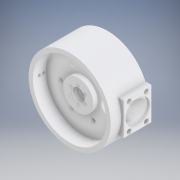
# Autodesk Inventor part: AA036
Saved by Autodesk Inventor 2017 SP1 (Build 210196100, 196)
## iProperties
Created: 2017-10-30
Part Number: AA036
Material: ABS Plastic
Document SubType Name: Modeling
Designer: Zach
Density: 1.06 g/cm^3
Appearance: CR White
Author: Zach
Autodesk Inventor part; units mm, degrees
ref_plane "YZ Plane" through (0, 0, 0) normal (1, 0, 0) x (0, 1, 0)
ref_plane "XZ Plane" through (0, 0, 0) normal (0, 1, 0) x (-1, 0, 0)
ref_plane "XY Plane" through (0, 0, 0) normal (0, 0, 1) x (1, 0, 0)
sketch "Sketch1" plane through (0, 0, 0) normal (0, 0, 1) x (1, 0, 0)
  circle A0 centre (0, 0) radius 47.5
  circle A1 centre (0, 0) radius 4.25
  circle A2 centre (25, 0) radius 2.5
  circle A3 centre (12.5, 21.6506) radius 2.5
  circle A4 centre (-12.5, 21.6506) radius 2.5
  circle A5 centre (-25, 0) radius 2.5
  circle A6 centre (-12.5, -21.6506) radius 2.5
  circle A7 centre (12.5, -21.6506) radius 2.5
  dimension "d0" = 95
  dimension "d1" = 8.5
  dimension "d2" = 5
  dimension "d3" = 25
  dimension "d6" = 360
  constraints: 8 centre point, 2 coincident, 1 horizontal alignment, 13 other
  measures "d0" diameter of A0
  measures "d1" diameter of A1
  measures "d2" diameter of A2
  measures "d3" distance of A2.centre point (0, 0)
extrude "Extrusion1" add sketch "Sketch1" along normal blind 54
ref_plane "Work Plane1" through (0, 0, 16) normal (0, 0, 1) x (1, 0, 0)
sketch "Sketch2" plane through (0, 0, 16) normal (0, 0, 1) x (1, 0, 0)
  circle A0 centre (0, 0) radius 47.5 projected
  line L0 (43.6427, 18.75) -> (50.6427, 18.75)
  line L1 (50.6427, 18.75) -> (50.6427, -18.75)
  line L2 (50.6427, -18.75) -> (43.6427, -18.75)
  line L3 (43.6427, -18.75) -> (43.6427, 18.75)
  point P0 (43.6427, 0)
  dimension "d11" = 7
  dimension "d12" = 37.5
  constraints: 8 end point, 2 parallel, 2 point on circle, 1 horizontal, 1 horizontal alignment, 1 midpoint, 1 perpendicular
  measures "d11" distance of L1.end L2.end
  measures "d12" distance of L0.end L1.end
extrude "Extrusion2" add sketch "Sketch2" along normal mid plane 32 contours A0 L0 L1 L2
sketch "Sketch3" plane through (50.6427, -18.75, 32) normal (1, 0, 0) x (0, 0, -1)
  line L0 (-14, 48.75) -> (46, 48.75)
  line L1 (46, 48.75) -> (46, -11.25)
  line L2 (46, -11.25) -> (-14, -11.25)
  line L3 (-14, -11.25) -> (-14, 48.75)
  line L4 (32, 37.5) -> (0, 37.5) projected
  line L5 (0, 0) -> (0, 37.5) projected
  line L6 (32, 0) -> (0, 0) projected
  line L7 (32, 37.5) -> (32, 0) projected
  line L8 (32, 37.5) -> (32, 0) projected
  point P0 (32, 18.75)
  point P1 (-14, 18.75)
  point P2 (32, 18.75)
  point P3 (16, 48.75)
  point P4 (16, 37.5)
  dimension "d15" = 60
  dimension "d16" = 60
  constraints: 8 end point, 4 midpoint, 2 parallel, 1 horizontal, 1 horizontal alignment, 1 perpendicular, 1 vertical alignment
  measures "d15" distance of L1.end L2.end
  measures "d16" distance of L0.end L1.end
extrude "Extrusion3" add sketch "Sketch3" along normal blind 10 contours L0 L1 L2 L3 | L7 L6 L5 L4
fillet "Fillet1" radius 20 4 edges at (55.6427, 30, 46) (55.6427, 30, -14) (55.6427, -30, -14) (55.6427, -30, 46)
sketch "Sketch4" plane through (60.6427, -18.75, 32) normal (1, 0, 0) x (0, 0, -1)
  line L0 (6, 33.75) -> (26, 33.75) construction
  line L1 (26, 33.75) -> (26, 3.75) construction
  line L2 (26, 3.75) -> (6, 3.75) construction
  line L3 (6, 3.75) -> (6, 33.75) construction
  line L4 (26, 48.75) -> (6, 48.75) projected
  line L5 (46, 8.75) -> (46, 28.75) projected
  circle A0 centre (6, 33.75) radius 2.5
  circle A1 centre (26, 33.75) radius 2.5
  circle A2 centre (6, 3.75) radius 2.5
  circle A3 centre (26, 3.75) radius 2.5
  point P0 (32, 18.75)
  point P1 (26, 18.75)
  point P2 (46, 18.75)
  point P3 (16, 33.75)
  point P4 (16, 48.75)
  dimension "d20" = 20
  dimension "d21" = 30
  dimension "d22" = 5
  dimension "d23" = 5
  dimension "d24" = 5
  dimension "d25" = 5
  constraints: 8 end point, 4 centre point, 4 coincident, 4 midpoint, 2 parallel, 1 horizontal, 1 horizontal alignment, 1 perpendicular, 1 vertical alignment
  measures "d20" distance of L1.end L2.end
  measures "d21" distance of L0.end L1.end
  measures "d22" diameter of A0
  measures "d23" diameter of A1
  measures "d24" diameter of A2
  measures "d25" diameter of A3
extrude "Extrusion4" cut sketch "Sketch4" against normal blind 35
sketch "Sketch5" plane through (60.6427, -18.75, 32) normal (1, 0, 0) x (0, 0, -1)
  circle A0 centre (16, 18.75) radius 14
  line L0 (46, 8.75) -> (46, 28.75) projected
  line L1 (6, -11.25) -> (26, -11.25) projected
  point P0 (32, 18.75)
  point P1 (16, -11.25)
  point P2 (46, 18.75)
  dimension "d28" = 28
  constraints: 2 midpoint, 1 centre point, 1 horizontal alignment, 1 vertical alignment
  measures "d28" diameter of A0
extrude "Extrusion5" cut sketch "Sketch5" against normal blind 13
sketch "Sketch6" plane through (0, 0, 54) normal (0, 0, 1) x (1, 0, 0)
  circle A0 centre (0, 0) radius 47.5 projected
extrude "Extrusion6" cut sketch "Sketch6" against normal blind 10
sketch "Sketch7" plane through (0, 0, 44) normal (0, 0, 1) x (1, 0, 0)
  circle A0 centre (0, 0) radius 47.5 projected
  circle A1 centre (0, 0) radius 42.5
  circle A2 centre (0, 0) radius 17.5
  dimension "d33" = 5
  dimension "d34" = 35
  constraints: 2 centre point, 1 coincident
  measures "d33" radial gap between concentric circles of A0 A1
  measures "d34" diameter of A2
extrude "Extrusion7" cut sketch "Sketch7" against normal blind 15 contours A1
sketch "Sketch8" plane through (0, 0, 44) normal (0, 0, 1) x (1, 0, 0)
  circle A0 centre (0, 0) radius 13.5
  dimension "d37" = 27
  constraints: 1 centre point, 1 coincident
  measures "d37" diameter of A0
extrude "Extrusion8" cut sketch "Sketch8" against normal blind 10
sketch "Sketch9" plane through (0, 0, 34) normal (0, 0, 1) x (1, 0, 0)
  circle A0 centre (0, 9.525) radius 1.5
  circle A1 centre (-8.2489, 4.7625) radius 1.5
  circle A2 centre (-8.2489, -4.7625) radius 1.5
  circle A3 centre (0, -9.525) radius 1.5
  circle A4 centre (8.2489, -4.7625) radius 1.5
  circle A5 centre (8.2489, 4.7625) radius 1.5
  point P0 (0, 0)
  dimension "d40" = 3
  dimension "d41" = 9.525
  dimension "d44" = 360
  constraints: 6 centre point, 1 vertical alignment, 13 other
  measures "d40" diameter of A0
  measures "d41" distance of A0.centre point (0, 0)
extrude "Extrusion9" cut sketch "Sketch9" against normal blind 15
sketch "Sketch10" plane through (0, 0, 0) normal (1, 0, 0) x (0, 1, 0)
  line L0 (-13.5, 34) -> (13.5, 34) projected
  line L1 (-13.5, 44) -> (13.5, 44) projected
  circle A0 centre (0, 36.75) radius 1.5
  circle A1 centre (0, 31.65) radius 1.5
  line L2 (-13.5, 34) -> (13.5, 34) projected
  line L3 (0, 34) -> (0, 35.25)
  line L4 (0, 35.25) -> (0, 33.15)
  point P0 (0, 0)
  point P1 (0, 38.25)
  dimension "d49" = 3
  dimension "d48" = 3
  dimension "d52" = 1.25
  dimension "d62" = 2.1
  constraints: 4 end point, 4 vertical alignment, 2 midpoint, 2 point on circle, 1 centre point, 1 perpendicular, 1 vertical, 2 other
  measures "d48" diameter of A0
  measures "d52" distance of L3.start L3.end
  measures "d62" distance of L3.end L4.end
extrude "Extrusion10" cut sketch "Sketch10" against normal through all
sketch "Sketch11" plane through (50.6427, -18.75, 32) normal (-1, 0, 0) x (0, 0, 1)
  line L0 (-96.7712, -90.236) -> (51.8699, -90.236)
  line L1 (51.8699, -90.236) -> (51.8699, 135.8944)
  line L2 (51.8699, 135.8944) -> (-96.7712, 135.8944)
  line L3 (-96.7712, 135.8944) -> (-96.7712, -90.236)
  point P0 (-32, 18.75)
  constraints: 8 end point, 2 parallel, 1 horizontal, 1 perpendicular
extrude "Extrusion11" cut sketch "Sketch11" against normal through all
sketch "Sketch12" plane through (0, 0, 34) normal (0, 0, 1) x (1, 0, 0)
  circle A0 centre (0, 0) radius 17.5 projected
extrude "Extrusion12" cut sketch "Sketch12" along normal through all
sketch "Sketch13" plane through (0, 0, 34) normal (0, 0, 1) x (1, 0, 0)
  circle A0 centre (0, 0) radius 7.5
  dimension "d59" = 15
  constraints: 1 centre point, 1 coincident
  measures "d59" diameter of A0
extrude "Extrusion13" cut sketch "Sketch13" against normal blind 5
ref_plane "Work Plane2" through (0, 0, 16) normal (0, 0, 1) x (1, 0, 0)
sketch "Sketch17" plane through (0, 0, 29) normal (0, 0, 1) x (1, 0, 0)
  line L0 (50.6427, 12.5) -> (50.6427, 17.5) projected
  line L1 (25.6427, 17.5) -> (25.6427, 12.5) projected
  line L2 (50.6427, -17.5) -> (50.6427, -12.5) projected
  line L3 (25.6427, -12.5) -> (25.6427, -17.5) projected
  line L4 (31.6427, 19.5) -> (36.6427, 19.5)
  line L5 (36.6427, 19.5) -> (36.6427, 10.5)
  line L6 (36.6427, 10.5) -> (31.6427, 10.5)
  line L7 (31.6427, 10.5) -> (31.6427, 19.5)
  line L8 (31.6427, -10.5) -> (36.6427, -10.5)
  line L9 (36.6427, -10.5) -> (36.6427, -19.5)
  line L10 (36.6427, -19.5) -> (31.6427, -19.5)
  line L11 (31.6427, -19.5) -> (31.6427, -10.5)
  point P0 (0, 0)
  point P1 (31.6427, 15)
  point P2 (25.6427, 15)
  point P3 (25.6427, -15)
  point P4 (31.6427, -15)
  dimension "d74" = 5
  dimension "d75" = 9
  dimension "d76" = 5
  dimension "d77" = 9
  dimension "d78" = 6
  constraints: 16 end point, 4 midpoint, 4 parallel, 2 horizontal, 2 horizontal alignment, 2 perpendicular, 1 vertical alignment
  measures "d74" distance of L5.end L6.end
  measures "d75" distance of L4.end L5.end
  measures "d76" distance of L9.end L10.end
  measures "d77" distance of L8.end L9.end
  measures "d78" distance between parallel lines of L1 L7
extrude "Extrusion17" cut sketch "Sketch17" against normal blind 8
sketch "Sketch19" plane through (0, 0, 0) normal (0, 0, -1) x (-1, 0, 0)
  line L0 (-31.6427, -10.5) -> (-36.6427, -10.5) projected
  line L1 (-31.6427, -19.5) -> (-31.6427, -10.5) projected
  line L2 (-36.6427, -19.5) -> (-31.6427, -19.5) projected
  line L3 (-36.6427, -10.5) -> (-36.6427, -19.5) projected
  line L4 (-31.6427, 19.5) -> (-36.6427, 19.5) projected
  line L5 (-31.6427, 10.5) -> (-31.6427, 19.5) projected
  line L6 (-36.6427, 10.5) -> (-31.6427, 10.5) projected
  line L7 (-36.6427, 19.5) -> (-36.6427, 10.5) projected
  point P0 (0, 0)
extrude "Extrusion18" cut sketch "Sketch19" against normal blind 11
ref_plane "Work Plane3" through (50.6427, -18.75, 32) normal (-0.7071068, 0, 0.7071068) x (0, 1, 0)
sketch "Sketch20" plane through (50.6427, -18.75, 32) normal (-0.7071068, 0, 0.7071068) x (0, 1, 0)
  circle A0 centre (18.75, 12.75) radius 10
  line L0 (18.75, 4.2426) -> (18.75, 4.2426)
  line L1 (0, 0) -> (37.5, 0) projected
  point P0 (18.75, 58.4372)
  point P1 (18.75, 0)
  dimension "d84" = 20
  dimension "d90" = 12.75
  constraints: 2 end point, 2 midpoint, 2 vertical alignment, 1 centre point
  measures "d84" diameter of A0
  measures "d90" distance of point (18.75, 0) A0.centre
extrude "Extrusion19" cut sketch "Sketch20" along normal blind 20 and the other way blind 19
body "Solid1"
